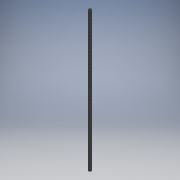
# Autodesk Inventor part: carbon_pipe
Saved by Autodesk Inventor 2017 (Build 210142000, 142)
## iProperties
Created: 2019-02-08
Part Number: carbon_pipe
Material: CFRP
Document SubType Name: Modeling
Designer: felix
Density: 1.43 g/cm^3
Appearance: Carbon Fiber
Author: felix
Autodesk Inventor part; units mm, degrees
ref_plane "YZ Plane" through (0, 0, 0) normal (1, 0, 0) x (0, 1, 0)
ref_plane "XZ Plane" through (0, 0, 0) normal (0, 1, 0) x (-1, 0, 0)
sketch "Sketch1" plane through (0, 0, 0) normal (0, 0, 1) x (1, 0, 0)
  circle A0 centre (0, 0) radius 4
  circle A1 centre (0, 0) radius 3
  dimension "d0" = 8
  dimension "d1" = 6
  constraints: 2 centre point, 2 coincident
  measures "d0" diameter of A0
  measures "d1" diameter of A1
extrude "Extrusion1" add sketch "Sketch1" along normal blind 414
ref_plane "Work Plane1" through (0, 0, 207) normal (0, 0, 1) x (1, 0, 0)
body "Solid1"
